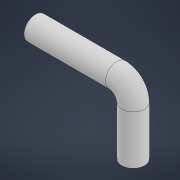
# Autodesk Inventor part: Pipe3
Saved by Autodesk Inventor 2022 (Build 260153070, 153G)
## iProperties
Created: 2021-07-21
Part Number: Pipe3
Material: Generic
Document SubType Name: Modeling
Designer: Eakawit_kor
Density: 1 g/cm^3
Appearance: Default
Author: Eakawit_kor
Autodesk Inventor part; units mm, degrees
ref_plane "YZ Plane" through (0, 0, 0) normal (1, 0, 0) x (0, 1, 0)
ref_plane "XZ Plane" through (0, 0, 0) normal (0, 1, 0) x (-1, 0, 0)
ref_plane "XY Plane" through (0, 0, 0) normal (0, 0, 1) x (1, 0, 0)
sketch "Sketch2" plane through (0, 0, 0) normal (1, 0, 0) x (0, 1, 0)
  circle A0 centre (0, 0) radius 1.5
  circle A1 centre (0, 0) radius 3.5
  dimension "d8" = 3
  dimension "d9" = 2
  constraints: 2 centre point, 1 coincident
  measures "d8" diameter of A0
  measures "d9" radial gap between concentric circles of A1 A0
sketch3d "3D Sketch1"
  line L0 (0, 0, 0) -> (25, 0, 0)
  arc A0 (25, 0, 0) -> (30, -5, 0) centre (25, -5, 0) ccw
  line L1 (30, -5, 0) -> (30, -20, 0)
  dimension "d3" = 30
  dimension "d4" = 20
  dimension "d6" = 5
sweep "Sweep1" add profiles "Sketch2" path "3D Sketch1"
body "Solid1"
